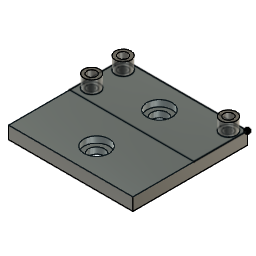
endstopMount (Autodesk Fusion 360 design; units mm, degrees)
Autodesk Fusion 360 part; units mm, degrees
sketch "Schizzo1" plane through (0, 0, 0) normal (0, 0, 1) x (1, 0, 0)
  line L0 (0, 0) -> (39.5, 0)
  line L1 (39.5, 0) -> (39.5, 36.4)
  line L2 (39.5, 36.4) -> (0, 36.4)
  line L3 (0, 36.4) -> (0, 0)
  dimension "d1" = 39.5
  dimension "d2" = 36.4
  constraint horizontal L0
  constraint vertical L1
  constraint horizontal L2
  constraint vertical L3
  constraint coincident L0.start L3.end
  measures "d1" distance of L0.start L0.end
  measures "d2" distance of L0.start L2.end
extrude "Estrusione1" add sketch "Schizzo1" along normal blind 4
sketch "Schizzo2" plane through (0, 0, 4) normal (0, 0, 1) x (-1, 0, 0)
  line L0 (0, -36.4) -> (0, 0)
  line L1 (0, 0) -> (-39.5, 0)
  line L2 (-39.5, 0) -> (-39.5, -36.4)
  line L3 (-39.5, -36.4) -> (0, -36.4)
  circle A0 centre (-19.75, -8.2) radius 2.55
  circle A1 centre (-19.75, -28.2) radius 2.55
  circle A2 centre (-19.75, -8.2) radius 4
  circle A3 centre (-19.75, -28.2) radius 4
  dimension "d5" = 5.1
  dimension "d6" = 5.1
  dimension "d7" = 8.2
  dimension "d8" = 19.75
  dimension "d9" = 8.2
  dimension "d10" = 19.75
  dimension "d11" = 8
  dimension "d12" = 8
  constraint concentric A0 A2
  constraint concentric A1 A3
  measures "d5" diameter of A0
  measures "d6" diameter of A1
  measures "d7" distance of L1 A0.centre
  measures "d8" distance of L0 A0.centre
  measures "d9" distance of L3 A1.centre
  measures "d10" distance of L0 A1.centre
  measures "d11" diameter of A2
  measures "d12" diameter of A3
extrude "Estrusione2" cut sketch "Schizzo2" against normal up to surface (4 mm away) contours A0
extrude "Estrusione3" cut sketch "Schizzo2" against normal up to surface (4 mm away) contours A1
extrude "Estrusione4" cut sketch "Schizzo2" against normal blind 2 contours A2 | A3
sketch "Schizzo3" plane through (0, 0, 4) normal (0, 0, 1) x (-1, 0, 0)
  circle A0 centre (-19.75, -8.2) radius 4
  circle A1 centre (-19.75, -28.2) radius 4
  line L0 (0, -36.4) -> (0, 0)
  line L1 (0, 0) -> (-39.5, 0)
  line L2 (-39.5, 0) -> (-39.5, -36.4)
  line L3 (-39.5, -36.4) -> (0, -36.4)
  line L4 (-39.5, -36.4) -> (0, -36.4)
  line L5 (0, -36.4) -> (0, -19.4)
  line L6 (0, -19.4) -> (-39.5, -19.4)
  line L7 (-39.5, -19.4) -> (-39.5, -36.4)
  circle A2 centre (-3, -23.4) radius 1.5
  circle A3 centre (-3, -33.4) radius 1.5
  circle A4 centre (-36.5, -33.4) radius 1.5
  circle A5 centre (-36.5, -33.4) radius 2.5
  circle A6 centre (-3, -33.4) radius 2.5
  circle A7 centre (-3, -23.4) radius 2.5
  dimension "d19" = 39.5
  dimension "d20" = 17
  dimension "d21" = 3
  dimension "d22" = 13
  dimension "d23" = 3
  dimension "d24" = 3
  dimension "d25" = 3
  dimension "d26" = 3
  dimension "d27" = 3
  dimension "d28" = 3
  dimension "d29" = 3
  dimension "d30" = 5
  dimension "d31" = 5
  dimension "d32" = 5
  constraint horizontal L4
  constraint vertical L5
  constraint horizontal L6
  constraint vertical L7
  constraint coincident L2.end L3.start
  constraint concentric A4 A5
  constraint concentric A3 A6
  constraint concentric A2 A7
  measures "d19" distance of L2.end L0.start
  measures "d20" distance of L2.end L6.end
  measures "d21" diameter of A2
  measures "d22" distance of L4 A2.centre
  measures "d23" diameter of A3
  measures "d24" distance of L4 A3.centre
  measures "d25" distance of L5 A3.centre
  measures "d26" distance of L5 A2.centre
  measures "d27" diameter of A4
  measures "d28" distance of L4 A4.centre
  measures "d29" distance of L7 A4.centre
  measures "d30" diameter of A5
  measures "d31" diameter of A6
  measures "d32" diameter of A7
extrude "Estrusione5" add sketch "Schizzo3" along normal blind 4 contours A5 | A6 | A7
